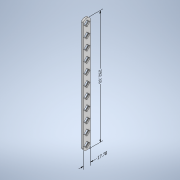
# Autodesk Inventor part: bar5
Saved by Autodesk Inventor 2020 (Build 240168000, 168)
## iProperties
Created: 2020-04-30
Part Number: bar5
Material: Generic
Document SubType Name: Modeling
Designer: alejandrosalazar
Density: 1 g/cm^3
Appearance: Default
Author: alejandrosalazar
Autodesk Inventor part; units mm, degrees
ref_plane "YZ Plane" through (0, 0, 0) normal (1, 0, 0) x (0, 1, 0)
ref_plane "XZ Plane" through (0, 0, 0) normal (0, 1, 0) x (-1, 0, 0)
ref_plane "XY Plane" through (0, 0, 0) normal (0, 0, 1) x (1, 0, 0)
sketch "Sketch1" plane through (0, 0, 0) normal (1, 0, 0) x (0, 1, 0)
  line L0 (0, 0) -> (292.1, 0)
  line L1 (292.1, 0) -> (292.1, -17.78)
  line L2 (292.1, -17.78) -> (0, -17.78)
  line L3 (0, -17.78) -> (0, 0)
  dimension "d0" = 292.1
  dimension "d1" = 17.78
  constraints: 8 end point, 2 parallel, 1 horizontal, 1 perpendicular
  measures "d0" distance of L1.end L2.end
  measures "d1" distance of L0.end L1.end
extrude "Extrusion1" add sketch "Sketch1" along normal blind 5
sketch "Sketch2" plane through (5, 0, 0) normal (1, 0, 0) x (0, 0, -1)
  line L0 (8.89, 273.81) -> (2.17, 280.53)
  line L1 (2.17, 280.53) -> (8.89, 287.25)
  line L2 (8.89, 287.25) -> (15.61, 280.53)
  line L3 (15.61, 280.53) -> (8.89, 273.81)
  line L4 (8.89, 246.794) -> (2.17, 253.514)
  line L5 (2.17, 253.514) -> (8.89, 260.234)
  line L6 (8.89, 260.234) -> (15.61, 253.514)
  line L7 (15.61, 253.514) -> (8.89, 246.794)
  line L8 (8.89, 219.928) -> (2.17, 226.648)
  line L9 (2.17, 226.648) -> (8.89, 233.368)
  line L10 (8.89, 233.368) -> (15.61, 226.648)
  line L11 (15.61, 226.648) -> (8.89, 219.928)
  line L12 (8.89, 193.062) -> (2.17, 199.782)
  line L13 (2.17, 199.782) -> (8.89, 206.502)
  line L14 (8.89, 206.502) -> (15.61, 199.782)
  line L15 (15.61, 199.782) -> (8.89, 193.062)
  line L16 (8.89, 166.196) -> (2.17, 172.916)
  line L17 (2.17, 172.916) -> (8.89, 179.636)
  line L18 (8.89, 179.636) -> (15.61, 172.916)
  line L19 (15.61, 172.916) -> (8.89, 166.196)
  line L20 (8.89, 139.33) -> (2.17, 146.05)
  line L21 (2.17, 146.05) -> (8.89, 152.77)
  line L22 (8.89, 152.77) -> (15.61, 146.05)
  line L23 (15.61, 146.05) -> (8.89, 139.33)
  line L24 (8.89, 112.464) -> (2.17, 119.184)
  line L25 (2.17, 119.184) -> (8.89, 125.904)
  line L26 (8.89, 125.904) -> (15.61, 119.184)
  line L27 (15.61, 119.184) -> (8.89, 112.464)
  line L28 (8.89, 85.598) -> (2.17, 92.318)
  line L29 (2.17, 92.318) -> (8.89, 99.038)
  line L30 (8.89, 99.038) -> (15.61, 92.318)
  line L31 (15.61, 92.318) -> (8.89, 85.598)
  line L32 (8.89, 58.732) -> (2.17, 65.452)
  line L33 (2.17, 65.452) -> (8.89, 72.172)
  line L34 (8.89, 72.172) -> (15.61, 65.452)
  line L35 (15.61, 65.452) -> (8.89, 58.732)
  line L36 (8.89, 31.866) -> (2.17, 38.586)
  line L37 (2.17, 38.586) -> (8.89, 45.306)
  line L38 (8.89, 45.306) -> (15.61, 38.586)
  line L39 (15.61, 38.586) -> (8.89, 31.866)
  line L40 (8.89, 5) -> (2.32, 11.57)
  line L41 (2.32, 11.57) -> (8.89, 18.14)
  line L42 (8.89, 18.14) -> (15.46, 11.57)
  line L43 (15.46, 11.57) -> (8.89, 5)
  point P0 (0, 0)
  point P1 (8.89, 280.53)
  point P2 (8.89, 253.514)
  point P3 (8.89, 226.648)
  point P4 (8.89, 199.782)
  point P5 (8.89, 172.916)
  point P6 (8.89, 146.05)
  point P7 (8.89, 119.184)
  point P8 (8.89, 92.318)
  point P9 (8.89, 65.452)
  point P10 (8.89, 38.586)
  point P11 (8.89, 11.57)
  constraints: 88 end point, 99 other
extrude "Extrusion2" cut sketch "Sketch2" against normal blind 5
fillet "Fillet1" radius 7 4 edges at (2.5, 292.1, 0) (2.5, 292.1, -17.78) (2.5, 0, 0) (2.5, 0, -17.78)
chamfer "Chamfer1" distance 1 distance2 2 1 edges at (5, 277.17, -12.25) measured on face at (5, 128.1393, -0.7233)
chamfer "Chamfer2" distance 1 distance2 2 1 edges at (5, 283.89, -5.53) measured on face at (5, 128.1393, -0.7233)
chamfer "Chamfer3" distance 1 distance2 2 1 edges at (5, 283.89, -12.25) measured on face at (5, 128.1393, -0.7233)
chamfer "Chamfer4" distance 1 distance2 2 1 edges at (5, 277.17, -5.53) measured on face at (5, 128.1393, -0.7233)
chamfer "Chamfer5" distance 1 distance2 2 1 edges at (0, 283.89, -5.53) measured on face at (0, 128.1393, -0.7233)
chamfer "Chamfer6" distance 1 distance2 2 1 edges at (0, 283.89, -12.25) measured on face at (0, 128.1393, -0.7233)
chamfer "Chamfer7" distance 1 distance2 2 1 edges at (0, 277.17, -12.25) measured on face at (0, 128.1393, -0.7233)
chamfer "Chamfer8" distance 1 distance2 2 1 edges at (0, 277.17, -5.53) measured on face at (0, 128.1393, -0.7233)
chamfer "Chamfer9" distance 1 distance2 2 1 edges at (0, 256.874, -12.25) measured on face at (0, 128.1393, -0.7233)
chamfer "Chamfer10" distance 1 distance2 2 1 edges at (0, 256.874, -5.53) measured on face at (0, 128.1393, -0.7233)
chamfer "Chamfer11" distance 1 distance2 2 1 edges at (0, 250.154, -12.25) measured on face at (0, 146.05, -17.0567)
chamfer "Chamfer12" distance 1 distance2 2 1 edges at (0, 250.154, -5.53) measured on face at (0, 135.5213, -16.8047)
chamfer "Chamfer13" distance 1 distance2 2 1 edges at (0, 230.008, -12.25) measured on face at (0, 135.5213, -16.8047)
chamfer "Chamfer14" distance 1 distance2 2 1 edges at (0, 230.008, -5.53) measured on face at (0, 135.5213, -16.8047)
chamfer "Chamfer15" distance 1 distance2 2 1 edges at (0, 223.288, -12.25) measured on face at (0, 135.5213, -16.8047)
chamfer "Chamfer16" distance 1 distance2 2 1 edges at (0, 223.288, -5.53) measured on face at (0, 117.6107, -16.8047)
chamfer "Chamfer17" distance 1 distance2 2 1 edges at (0, 203.142, -12.25) measured on face at (0, 117.6107, -16.8047)
chamfer "Chamfer18" distance 1 distance2 2 1 edges at (0, 196.422, -12.25) measured on face at (0, 117.6107, -16.8047)
chamfer "Chamfer19" distance 1 distance2 2 1 edges at (0, 203.142, -5.53) measured on face at (0, 108.6553, -16.8047)
chamfer "Chamfer20" distance 1 distance2 2 1 edges at (0, 196.422, -5.53) measured on face at (0, 108.6553, -16.8047)
chamfer "Chamfer21" distance 1 distance2 2 1 edges at (0, 176.276, -12.25) measured on face at (0, 108.6553, -16.8047)
chamfer "Chamfer22" distance 1 distance2 2 1 edges at (0, 169.556, -5.53) measured on face at (0, 126.566, -0.9753)
chamfer "Chamfer23" distance 1 distance2 2 1 edges at (0, 176.276, -5.53) measured on face at (0, 172.916, -0.2519)
chamfer "Chamfer24" distance 1 distance2 2 1 edges at (0, 169.556, -12.25) measured on face at (0, 108.6553, -0.9753)
chamfer "Chamfer25" distance 1 distance2 2 1 edges at (0, 149.41, -5.53) measured on face at (0, 90.7447, -16.8047)
chamfer "Chamfer26" distance 1 distance2 2 1 edges at (0, 149.41, -12.25) measured on face at (0, 90.7447, -16.8047)
chamfer "Chamfer27" distance 1 distance2 2 1 edges at (0, 142.69, -12.25) measured on face at (0, 155.0053, -0.2519)
chamfer "Chamfer28" distance 1 distance2 2 1 edges at (0, 142.69, -5.53) measured on face at (0, 81.7893, -16.8047)
chamfer "Chamfer29" distance 1 distance2 2 1 edges at (0, 122.544, -12.25) measured on face at (0, 81.7893, -16.8047)
chamfer "Chamfer30" distance 1 distance2 2 1 edges at (0, 122.544, -5.53) measured on face at (0, 90.7447, -0.9753)
chamfer "Chamfer31" distance 1 distance2 2 1 edges at (0, 115.824, -12.25) measured on face at (0, 146.05, -0.2519)
chamfer "Chamfer32" distance 1 distance2 2 1 edges at (0, 115.824, -5.53) measured on face at (0, 146.05, -0.2519)
chamfer "Chamfer33" distance 1 distance2 2 1 edges at (0, 95.678, -12.25) measured on face at (0, 146.05, -0.2519)
chamfer "Chamfer34" distance 1 distance2 2 1 edges at (0, 95.678, -5.53) measured on face at (0, 146.05, -0.2519)
chamfer "Chamfer35" distance 1 distance2 2 1 edges at (0, 88.958, -12.25) measured on face at (0, 146.05, -0.2519)
chamfer "Chamfer36" distance 1 distance2 2 1 edges at (0, 88.958, -5.53) measured on face at (0, 146.05, -0.2519)
chamfer "Chamfer37" distance 1 distance2 2 1 edges at (0, 68.812, -12.25) measured on face at (0, 146.05, -0.2519)
chamfer "Chamfer38" distance 1 distance2 2 1 edges at (0, 68.812, -5.53) measured on face at (0, 146.05, -0.2519)
chamfer "Chamfer39" distance 1 distance2 2 1 edges at (0, 62.092, -12.25) measured on face at (0, 146.05, -0.2519)
chamfer "Chamfer40" distance 1 distance2 2 1 edges at (0, 62.092, -5.53) measured on face at (0, 146.05, -0.2519)
chamfer "Chamfer41" distance 1 distance2 2 1 edges at (0, 41.946, -5.53) measured on face at (0, 146.05, -0.2519)
chamfer "Chamfer42" distance 1 distance2 2 1 edges at (0, 41.946, -12.25) measured on face at (0, 146.05, -0.2519)
chamfer "Chamfer43" distance 1 distance2 2 1 edges at (0, 35.226, -12.25) measured on face at (0, 146.05, -0.2519)
chamfer "Chamfer44" distance 1 distance2 2 1 edges at (0, 35.226, -5.53) measured on face at (0, 146.05, -0.2519)
chamfer "Chamfer45" distance 1 distance2 2 1 edges at (0, 8.285, -5.605) measured on face at (0, 146.05, -0.2519)
chamfer "Chamfer46" distance 1 distance2 2 1 edges at (0, 14.855, -5.605) measured on face at (0, 146.05, -0.2519)
chamfer "Chamfer47" distance 1 distance2 2 1 edges at (0, 14.855, -12.175) measured on face at (0, 146.05, -0.2519)
chamfer "Chamfer48" distance 1 distance2 2 1 edges at (0, 8.285, -12.175) measured on face at (0, 146.05, -0.2519)
chamfer "Chamfer49" distance 1 distance2 2 1 edges at (5, 256.874, -5.53) measured on face at (5, 128.1393, -0.7233)
chamfer "Chamfer50" distance 1 distance2 2 1 edges at (5, 256.874, -12.25) measured on face at (5, 146.05, -17.0567)
chamfer "Chamfer51" distance 1 distance2 2 1 edges at (5, 250.154, -5.53) measured on face at (5, 146.05, -17.0567)
chamfer "Chamfer52" distance 1 distance2 2 1 edges at (5, 250.154, -12.25) measured on face at (5, 146.05, -17.0567)
chamfer "Chamfer53" distance 1 distance2 2 1 edges at (5, 230.008, -5.53) measured on face at (5, 135.5213, -16.8047)
chamfer "Chamfer54" distance 1 distance2 2 1 edges at (5, 230.008, -12.25) measured on face at (5, 135.5213, -16.8047)
chamfer "Chamfer55" distance 1 distance2 2 1 edges at (5, 223.288, -5.53) measured on face at (5, 135.5213, -16.8047)
chamfer "Chamfer56" distance 1 distance2 2 1 edges at (5, 223.288, -12.25) measured on face at (5, 135.5213, -16.8047)
chamfer "Chamfer57" distance 1 distance2 2 1 edges at (5, 203.142, -5.53) measured on face at (5, 117.6107, -16.8047)
chamfer "Chamfer58" distance 1 distance2 2 1 edges at (5, 203.142, -12.25) measured on face at (5, 117.6107, -16.8047)
chamfer "Chamfer59" distance 1 distance2 2 1 edges at (5, 196.422, -5.53) measured on face at (5, 117.6107, -16.8047)
chamfer "Chamfer60" distance 1 distance2 2 1 edges at (5, 196.422, -12.25) measured on face at (5, 117.6107, -16.8047)
chamfer "Chamfer61" distance 1 distance2 2 1 edges at (5, 176.276, -5.53) measured on face at (5, 108.6552, -16.8046)
chamfer "Chamfer62" distance 1 distance2 2 1 edges at (5, 176.276, -12.25) measured on face at (5, 108.6552, -16.8046)
chamfer "Chamfer63" distance 1 distance2 2 1 edges at (5, 169.556, -5.53) measured on face at (5, 163.9605, -17.528)
chamfer "Chamfer64" distance 1 distance2 2 1 edges at (5, 169.556, -12.25) measured on face at (5, 108.6553, -0.9753)
chamfer "Chamfer65" distance 1 distance2 2 1 edges at (5, 149.41, -5.53) measured on face at (5, 90.7447, -16.8047)
chamfer "Chamfer66" distance 1 distance2 2 1 edges at (5, 149.41, -12.25) measured on face at (5, 90.7447, -16.8047)
chamfer "Chamfer67" distance 1 distance2 2 1 edges at (5, 142.69, -5.53) measured on face at (5, 155.0053, -17.5281)
chamfer "Chamfer68" distance 1 distance2 2 1 edges at (5, 142.69, -12.25) measured on face at (5, 90.7447, -0.9753)
chamfer "Chamfer69" distance 1 distance2 2 1 edges at (5, 122.544, -5.53) measured on face at (5, 81.7893, -16.8047)
chamfer "Chamfer70" distance 1 distance2 2 1 edges at (5, 122.544, -12.25) measured on face at (5, 81.7893, -16.8047)
chamfer "Chamfer71" distance 1 distance2 2 1 edges at (5, 115.824, -5.53) measured on face at (5, 146.05, -0.2519)
chamfer "Chamfer72" distance 1 distance2 2 1 edges at (5, 115.824, -12.25) measured on face at (5, 146.05, -0.2519)
chamfer "Chamfer73" distance 1 distance2 2 1 edges at (5, 95.678, -5.53) measured on face at (5, 146.05, -0.2519)
chamfer "Chamfer74" distance 1 distance2 2 1 edges at (5, 95.678, -12.25) measured on face at (5, 146.05, -0.2519)
chamfer "Chamfer75" distance 1 distance2 2 1 edges at (5, 88.958, -5.53) measured on face at (5, 146.05, -0.2519)
chamfer "Chamfer76" distance 1 distance2 2 1 edges at (5, 88.958, -12.25) measured on face at (5, 146.05, -0.2519)
chamfer "Chamfer77" distance 1 distance2 2 1 edges at (5, 68.812, -5.53) measured on face at (5, 146.05, -0.2519)
chamfer "Chamfer78" distance 1 distance2 2 1 edges at (5, 68.812, -12.25) measured on face at (5, 146.05, -0.2519)
chamfer "Chamfer79" distance 1 distance2 2 1 edges at (5, 62.092, -5.53) measured on face at (5, 146.05, -0.2519)
chamfer "Chamfer80" distance 1 distance2 2 1 edges at (5, 62.092, -12.25) measured on face at (5, 146.05, -0.2519)
chamfer "Chamfer81" distance 1 distance2 2 1 edges at (5, 41.946, -5.53) measured on face at (5, 146.05, -0.2519)
chamfer "Chamfer82" distance 1 distance2 2 1 edges at (5, 41.946, -12.25) measured on face at (5, 146.05, -0.2519)
chamfer "Chamfer83" distance 1 distance2 2 1 edges at (5, 35.226, -5.53) measured on face at (5, 146.05, -0.2519)
chamfer "Chamfer84" distance 1 distance2 2 1 edges at (5, 35.226, -12.25) measured on face at (5, 146.05, -0.2519)
chamfer "Chamfer85" distance 1 distance2 2 1 edges at (5, 14.855, -5.605) measured on face at (5, 146.05, -0.2519)
chamfer "Chamfer86" distance 1 distance2 2 1 edges at (5, 14.855, -12.175) measured on face at (5, 146.05, -0.2519)
chamfer "Chamfer87" distance 1 distance2 2 1 edges at (5, 8.285, -5.605) measured on face at (5, 146.05, -0.2519)
chamfer "Chamfer88" distance 1 distance2 2 1 edges at (5, 8.285, -12.175) measured on face at (5, 146.05, -0.2519)
body "Solid1"
